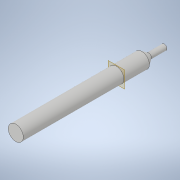
# Autodesk Inventor part: nozzle mould tool
Saved by Autodesk Inventor 2020.3 (Build 243373000, 373)
## iProperties
Created: 2021-04-26
Part Number: nozzle mould tool
Material: Generic
Document SubType Name: Modeling
Designer: Mike
Density: 1 g/cm^3
Appearance: Default
Author: Mike
Autodesk Inventor part; units mm, degrees
ref_plane "YZ Plane" through (0, 0, 0) normal (1, 0, 0) x (0, 1, 0)
ref_plane "XZ Plane" through (0, 0, 0) normal (0, 1, 0) x (-1, 0, 0)
sketch "Sketch1" plane through (0, 0, 0) normal (1, 0, 0) x (0, 1, 0)
  line L0 (0, 0) -> (15, 0)
  line L1 (0, 0) -> (5.5, 0)
  line L2 (0, 0) -> (11, 0)
  line L3 (15, -0.7141) -> (5.5, -14.2815)
  line L4 (15.5, 0) -> (35.4603, 0) construction
  line L5 (5.5, -14.2815) -> (5.5, -19.2815)
  line L6 (5.5, -19.2815) -> (11, -45.1569) construction
  line L7 (5.5, -19.2815) -> (64.4036, -19.2815) construction
  line L8 (0, 0) -> (11, 0)
  line L9 (11, 0) -> (11, -45.1569) construction
  line L10 (5.5, -19.2815) -> (5.5, -62.0623)
  line L11 (5.5, -45.1569) -> (0, -45.1569)
  line L12 (0, 0) -> (0, -45.1569)
  line L13 (0, -74.4747) -> (0, 12.4125) projected
  line L14 (0, 0) -> (15, 0)
  line L15 (15, 0) -> (15, -0.7141)
  line L16 (15, -19.2815) -> (15, -27.5658)
  dimension "d17" = 5.5
  dimension "d22" = 15.5
  dimension "d23" = 125
  dimension "d24" = 5
  dimension "d25" = 78
  dimension "d27" = 11
  dimension "d28" = 45.157
  dimension "d30" = 15
  constraints: 32 end point, 4 horizontal, 4 perpendicular, 4 point on line, 2 vertical, 1 collinear
  measures "d17" distance of L0.start L1.end
  measures "d22" distance of L0.start L4.start
  measures "d23" angle of L3 L4
  measures "d24" distance of L3.end L5.end
  measures "d25" angle of L6 L7
  measures "d27" distance of L0.start L2.end
  measures "d28" distance of L0.start L11.end
  measures "d30" distance of L0.end L0.start
revolve "Revolution2" add sketch "Sketch1" angle 360 about axis through (0, 0, -10) along (0, 0, 1)
sketch "Sketch2" plane through (0, 0, 0) normal (0, 0, 1) x (1, 0, 0)
  circle A0 centre (0, 0) radius 15
  dimension "d31" = 30
  constraints: 1 centre point, 1 coincident
  measures "d31" diameter of A0
extrude "Extrusion1" add sketch "Sketch2" along normal blind 250
ref_plane "Work Plane1" through (0, 0, 50) normal (0, 0, 1) x (1, 0, 0)
split body "Split1" result two bodies by plane through (0, 0, 50) normal (0, 0, 1) first body at (14.453, -1.1668, 183.3333)
body "Solid3"
body "Solid4"
